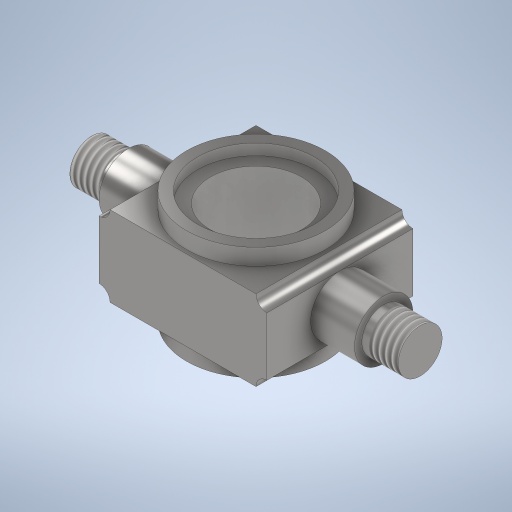
# Autodesk Inventor part: HookAnchor
Saved by Autodesk Inventor 2023.2 (Build 272271030, 271C)
## iProperties
Created: 2023-03-27
Part Number: HookAnchor
Material: Stainless Steel
Document SubType Name: Modeling
Designer: Luis Valente
Density: 8 g/cm^3
Appearance: Semi-Polished
Author: Luis Valente
Autodesk Inventor part; units mm, degrees
ref_plane "YZ Plane" through (0, 0, 0) normal (1, 0, 0) x (0, 1, 0)
ref_plane "XZ Plane" through (0, 0, 0) normal (0, 1, 0) x (-1, 0, 0)
ref_plane "XY Plane" through (0, 0, 0) normal (0, 0, 1) x (1, 0, 0)
sketch "Sketch7" plane through (0, 0, 0) normal (0, 1, 0) x (-1, 0, 0)
  circle A0 centre (0, 0) radius 19
  dimension "d19" = 38
  constraints: 1 centre point, 1 coincident
  measures "d19" diameter of A0
extrude "Extrusion7" add sketch "Sketch7" along normal mid plane 31
sketch "Sketch8" plane through (0, 15.5, 0) normal (0, 1, 0) x (1, 0, 0)
  circle A0 centre (0, 0) radius 16
  dimension "d22" = 32
  constraints: 1 centre point, 1 coincident
  measures "d22" diameter of A0
extrude "Extrusion8" cut sketch "Sketch8" against normal blind 3
sketch "Sketch9" plane through (0, -15.5, 0) normal (0, -1, 0) x (1, 0, 0)
  circle A0 centre (0, 0) radius 16
  dimension "d25" = 32
  constraints: 1 centre point, 1 coincident
  measures "d25" diameter of A0
extrude "Extrusion9" cut sketch "Sketch9" against normal blind 3
sketch "Sketch12" plane through (0, 0, 0) normal (0, 1, 0) x (-1, 0, 0)
  line L0 (-23, -20) -> (23, -20)
  line L1 (23, -20) -> (23, 20)
  line L2 (23, 20) -> (-23, 20)
  line L3 (-23, 20) -> (-23, -20)
  line L4 (-23, -20) -> (23, 20) construction
  line L5 (23, -20) -> (-23, 20) construction
  line L6 (-23, -20) -> (23, -20) construction
  point P0 (0, 0)
  dimension "d34" = 46
  dimension "d35" = 0
  dimension "d36" = 40
  constraints: 14 end point, 2 horizontal, 2 midpoint, 2 parallel, 1 collinear, 1 perpendicular
  measures "d34" distance of L0.start L0.end
  measures "d35" distance between parallel lines of L0 L6
  measures "d36" distance of L1.end L0.end
extrude "Extrusion11" add sketch "Sketch12" along normal mid plane 22
sketch "Sketch13" plane through (23, -11, -20) normal (1, 0, 0) x (0, 0, -1)
  circle A0 centre (-20, 11) radius 8
  dimension "d39" = 16
  constraints: 1 centre point, 1 coincident
  measures "d39" diameter of A0
extrude "Extrusion12" add sketch "Sketch13" along normal blind 12 and the other way blind 58
sketch "Sketch14" plane through (35, 0, 0) normal (1, 0, 0) x (0, 0, -1)
  circle A0 centre (0, 0) radius 6
  dimension "d44" = 12
  constraints: 1 centre point, 1 coincident
  measures "d44" diameter of A0
extrude "Extrusion13" add sketch "Sketch14" along normal blind 10
thread "Thread1" size "M12x1.75" class "6g" standard "ISO Metric profile" length 8
sketch "Sketch15" plane through (-35, 0, 0) normal (-1, 0, 0) x (0, 0, 1)
  circle A0 centre (0, 0) radius 6
  dimension "d49" = 12
  constraints: 1 centre point, 1 coincident
  measures "d49" diameter of A0
extrude "Extrusion14" add sketch "Sketch15" along normal blind 10
thread "Thread2" size "M12x1.75" class "6g" standard "ISO Metric profile" length 8
sketch "Sketch10" plane through (0, 12.5, 0) normal (0, 1, 0) x (1, 0, 0)
  circle A0 centre (0, 0) radius 12.5
  dimension "d28" = 25
  constraints: 1 centre point, 1 coincident
  measures "d28" diameter of A0
extrude "Extrusion10" cut sketch "Sketch10" against normal blind 31
fillet "Fillet1" radius 3 4 edges at (23, 11, 0) (-23, 11, 0) (-23, -11, 0) (23, -11, 0) inverted yes
body "Solid2"
